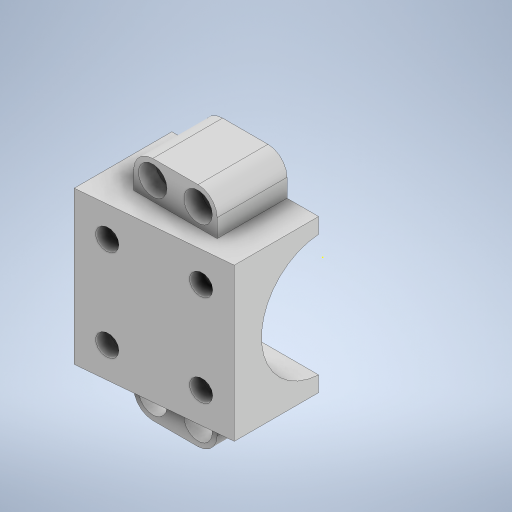
# Autodesk Inventor part: uchwyt
Saved by Autodesk Inventor 2023 (Build 270158000, 158)
## iProperties
Created: 2023-05-30
Part Number: uchwyt
Material: Ogólny
Document SubType Name: Modeling
Designer: Kamil
Density: 1 g/cm^3
Appearance: Domyślna
Author: Kamil
Autodesk Inventor part; units mm, degrees
ref_plane "YZ Plane" through (0, 0, 0) normal (1, 0, 0) x (0, 1, 0)
ref_plane "XZ Plane" through (0, 0, 0) normal (0, 1, 0) x (-1, 0, 0)
ref_plane "XY Plane" through (0, 0, 0) normal (0, 0, 1) x (1, 0, 0)
sketch "Szkic1" plane through (0, 0, 0) normal (0, 1, 0) x (-1, 0, 0)
  line L0 (-115.2766, 10.5) -> (-153.7841, 10.5)
  line L1 (-153.7841, 10.5) -> (-153.7841, 49.5698)
  line L2 (-153.7841, 49.5698) -> (-120, 49.5698)
  line L3 (-113.7841, 10.5) -> (-113.7841, 10.5489)
  line L4 (-19.8138, 58.6953) -> (-19.8138, 1.8047)
  line L5 (-19.8138, 58.6953) -> (-120, 49.5698)
  line L6 (-19.8138, 1.8047) -> (-115.2766, 10.5)
  point P0 (0, 0)
  constraints: 14 end point, 1 horizontal, 1 parallel, 1 perpendicular, 1 point on line, 1 vertical
extrude "Wyciągnięcie proste1" add sketch "Szkic1" along normal blind 40
sketch "Szkic2" plane through (0, 40, 0) normal (0, 1, 0) x (1, 0, 0)
  line L0 (120, -49.5698) -> (153.7841, -49.5698) projected
  line L1 (153.7841, -49.5698) -> (153.7841, -10.5) projected
  line L2 (153.7841, -10.5) -> (115.2766, -10.5) projected
  line L3 (115.2766, -10.5) -> (19.8138, -1.8047) projected
  line L4 (19.8138, -1.8047) -> (19.8138, -58.6953) projected
  line L5 (19.8138, -58.6953) -> (120, -49.5698) projected
  line L6 (19.8138, -30.25) -> (183, -30.25)
  point P0 (0, 0)
  point P1 (153.7841, -30.25)
  constraints: 2 end point, 1 horizontal, 1 midpoint
extrude "Wyciągnięcie proste2" cut sketch "Szkic2" against normal blind 40 contours L6 L4 L3 L2 L1
sketch "Szkic3" plane through (153.7841, 0, 49.5698) normal (1, 0, 0) x (0, 0, -1)
  line L0 (19.3198, 0) -> (19.3198, 40) projected
  line L1 (19.3198, 40) -> (19.3198, 0) projected
  circle A0 centre (19.3198, 20) radius 16
  point P0 (49.5698, 0)
  dimension "d4" = 32
  constraints: 1 centre point, 1 midpoint
  measures "d4" diameter of A0
extrude "Wyciągnięcie proste3" cut sketch "Szkic3" against normal through all
sketch "Szkic4" plane through (0, 40, 0) normal (0, 1, 0) x (1, 0, 0)
  line L0 (19.8138, -30.25) -> (19.8138, -58.6953) projected
  line L1 (19.8138, -30.25) -> (39.8138, -30.25)
  line L2 (39.8138, -30.25) -> (39.8138, -60.25)
  line L3 (39.8138, -60.25) -> (19.8138, -60.25)
  line L4 (19.8138, -60.25) -> (19.8138, -30.25)
  point P0 (0, 0)
  dimension "d7" = 20
  dimension "d8" = 30
  constraints: 8 end point, 2 parallel, 1 horizontal, 1 perpendicular
  measures "d7" distance of L2.end L3.end
  measures "d8" distance of L1.end L2.end
extrude "Wyciągnięcie proste4" cut sketch "Szkic4" against normal through all
sketch "Szkic5" plane through (120, 0, 49.5698) normal (0, 0, 1) x (1, 0, 0)
  line L0 (0, 40) -> (33.7841, 40) projected
  line L1 (0, 0) -> (0, 40) projected
  line L2 (33.7841, 40) -> (-80.1862, 40) projected
  line L3 (33.7841, 40) -> (0, 40)
  line L4 (33.7841, 36) -> (33.7841, 40) projected
  line L5 (33.7841, 40) -> (0, 40)
  line L6 (0, 40) -> (0, 52)
  line L7 (0, 52) -> (33.7841, 52)
  line L8 (33.7841, 52) -> (33.7841, 40)
  line L9 (0, 52) -> (5, 52)
  line L10 (5, 40) -> (0, 40)
  line L11 (0, 40) -> (0, 52)
  line L12 (33.7841, 52) -> (28.7841, 52)
  line L13 (28.7841, 40) -> (33.7841, 40)
  line L14 (33.7841, 40) -> (33.7841, 52)
  circle A0 centre (5, 44.75) radius 2.25
  circle A1 centre (28.7841, 44.75) radius 2.25
  circle A2 centre (16.8921, 44.75) radius 2.25
  circle A3 centre (5, 44.75) radius 5
  circle A4 centre (28.7841, 44.75) radius 5
  line L15 (5, 49.75) -> (28.7841, 49.75)
  point P0 (-120, 0)
  point P1 (0, 44.75)
  point P2 (33.7841, 44.75)
  dimension "d12" = 12
  dimension "d13" = 5
  dimension "d14" = 5
  constraints: 24 end point, 4 horizontal, 4 parallel, 3 centre point, 2 coincident, 2 point on line, 2 vertical, 1 collinear, 1 perpendicular, 6 other
  measures "d12" distance of L5.end L6.end
  measures "d13" distance of L10.start L10.end
  measures "d14" distance of L13.end L13.start
extrude "Wyciągnięcie proste5" add sketch "Szkic5" against normal up to surface (19.3198 mm away) contours L6 A3 L0 | A3 L0 | A3 L15 A4 L0 | A4 L0 | A4 L8 L0 picked at (4.3892, 40.8388) picked at (28.1733, 40.8388)
sketch "Szkic6" plane through (120, 0, 49.5698) normal (0, 0, 1) x (1, 0, 0)
  circle A0 centre (28.7841, 44.75) radius 2.25 projected
  circle A1 centre (16.8921, 44.75) radius 2.25 projected
  circle A2 centre (5, 44.75) radius 2.25 projected
  line L0 (0, 0) -> (33.7841, 0) projected
  line L1 (33.7841, 0) -> (33.7841, 44.75) projected
  arc A3 (33.7841, 44.75) -> (28.7841, 49.75) centre (28.7841, 44.75) ccw projected
  line L2 (28.7841, 49.75) -> (5, 49.75) projected
  arc A4 (5, 49.75) -> (0, 44.75) centre (5, 44.75) ccw projected
  line L3 (0, 44.75) -> (0, 40) projected
  line L4 (0, 0) -> (0, 40) projected
  line L5 (0, 40) -> (-80.1862, 40) projected
  line L6 (0, 40) -> (0, 0)
  line L7 (-80.1862, 0) -> (33.7841, 0) projected
  line L8 (0, 20) -> (40, 20)
  circle A5 centre (28.7841, -4.75) radius 2.25
  circle A6 centre (16.8921, -4.75) radius 2.25
  circle A7 centre (5, -4.75) radius 2.25
  line L9 (33.7841, 40) -> (33.7841, -4.75)
  arc A8 (28.7841, -9.75) -> (33.7841, -4.75) centre (28.7841, -4.75) ccw
  line L10 (28.7841, -9.75) -> (5, -9.75)
  arc A9 (0, -4.75) -> (5, -9.75) centre (5, -4.75) ccw
  line L11 (0, -4.75) -> (0, 0)
  point P0 (-120, 0)
  constraints: 10 end point, 10 symmetric about line, 5 centre point, 4 point on circle, 1 horizontal, 1 midpoint, 1 perpendicular, 5 other
extrude "Wyciągnięcie proste6" add sketch "Szkic6" against normal up to surface (19.3198 mm away) contours L0 L9 A8 L10 A9 L11
sketch "Szkic7" plane through (125, 49.75, 49.5698) normal (0, 0, 1) x (1, 0, 0)
  circle A0 centre (0, -54.5) radius 2.25 projected
  circle A1 centre (23.7841, -54.5) radius 2.25 projected
  circle A2 centre (11.8921, -54.5) radius 2.25 projected
  circle A3 centre (23.7841, -5) radius 2.25 projected
  circle A4 centre (11.8921, -5) radius 2.25 projected
  circle A5 centre (0, -5) radius 2.25 projected
  line L0 (28.7841, -54.5) -> (28.7841, -5) projected
  arc A6 (28.7841, -5) -> (23.7841, 0) centre (23.7841, -5) ccw projected
  line L1 (23.7841, 0) -> (0, 0) projected
  arc A7 (0, 0) -> (-5, -5) centre (0, -5) ccw projected
  line L2 (-5, -5) -> (-5, -9.75) projected
  line L3 (-5, -49.75) -> (-5, -9.75) projected
  line L4 (-5, -49.75) -> (-5, -54.5) projected
  arc A8 (-5, -54.5) -> (0, -59.5) centre (0, -54.5) ccw projected
  line L5 (0, -59.5) -> (23.7841, -59.5) projected
  arc A9 (23.7841, -59.5) -> (28.7841, -54.5) centre (23.7841, -54.5) ccw projected
  point P0 (-125, -49.75)
hole "Otwór1" at (125, 44.75, 49.5698) at (136.8921, 44.75, 49.5698) at (148.7841, 44.75, 49.5698) at (148.7841, -4.75, 49.5698) at (136.8921, -4.75, 49.5698) at (125, -4.75, 49.5698) direction (0, 0, -1) diameter 4.5 depth 40 tip angle 118 counterbore diameter 7.5 counterbore depth 4.5
sketch "Szkic8" plane through (125, 49.75, 49.5698) normal (0, 0, 1) x (1, 0, 0)
  circle A0 centre (11.8921, -54.5) radius 3.75 projected
  circle A1 centre (23.7841, -5) radius 3.75 projected
  circle A2 centre (0, -5) radius 3.75 projected
  circle A3 centre (11.8921, -5) radius 3.75 projected
  circle A4 centre (23.7841, -54.5) radius 3.75 projected
  circle A5 centre (0, -54.5) radius 3.75 projected
  line L0 (28.7841, -54.5) -> (28.7841, -5) projected
  arc A6 (28.7841, -5) -> (23.7841, 0) centre (23.7841, -5) ccw projected
  line L1 (23.7841, 0) -> (0, 0) projected
  arc A7 (0, 0) -> (-5, -5) centre (0, -5) ccw projected
  line L2 (-5, -5) -> (-5, -9.75) projected
  line L3 (-5, -49.75) -> (-5, -9.75) projected
  line L4 (-5, -49.75) -> (-5, -54.5) projected
  arc A8 (-5, -54.5) -> (0, -59.5) centre (0, -54.5) ccw projected
  line L5 (0, -59.5) -> (23.7841, -59.5) projected
  arc A9 (23.7841, -59.5) -> (28.7841, -54.5) centre (23.7841, -54.5) ccw projected
  line L6 (-85.1862, -9.75) -> (-85.1862, -49.75) projected
  circle A10 centre (0, -5) radius 2.25 projected
  line L7 (0, -5) -> (-30, -5)
  line L8 (-30, -5) -> (-30, -64)
  circle A11 centre (0, -54.5) radius 2.25 projected
  circle A12 centre (11.8921, -5) radius 2.25 projected
  circle A13 centre (11.8921, -54.5) radius 2.25 projected
  arc A14 (-55, -5) -> (-60, 0) centre (-60, -5) ccw
  line L9 (-55, -5) -> (-55, -9.75)
  line L10 (-55, -49.75) -> (-55, -9.75)
  line L11 (-55, -49.75) -> (-55, -54.5)
  arc A15 (-60, -59.5) -> (-55, -54.5) centre (-60, -54.5) ccw
  line L12 (-60, -59.5) -> (-71.8921, -59.5)
  arc A16 (-71.8921, 0) -> (-76.8921, -5) centre (-71.8921, -5) ccw
  arc A17 (-76.8921, -54.5) -> (-71.8921, -59.5) centre (-71.8921, -54.5) ccw
  line L13 (-76.8921, -5) -> (-76.8921, -54.5)
  line L14 (-71.8921, 0) -> (-60, 0)
  point P0 (-125, -49.75)
  point P1 (-83.7841, -59.5)
  dimension "d28" = 30
  constraints: 16 end point, 9 symmetric about line, 8 point on circle, 4 centre point, 3 tangent, 2 horizontal, 1 perpendicular, 2 other
  measures "d28" distance of L7.start L7.end
extrude "Wyciągnięcie proste7" add sketch "Szkic8" against normal up to surface (19.3198 mm away) contours L9 L10 L11 A15 L12 A17 L13 A16 L14 A14
sketch "Szkic9" plane through (125, 49.75, 49.5698) normal (0, 0, 1) x (1, 0, 0)
  line L0 (-55, -9.75) -> (-76.8921, -9.75) projected
  line L1 (-55, -9.75) -> (-55, -5) projected
  arc A0 (-55, -5) -> (-60, 0) centre (-60, -5) ccw projected
  line L2 (-60, 0) -> (-71.8921, 0) projected
  arc A1 (-71.8921, 0) -> (-76.8921, -5) centre (-71.8921, -5) ccw projected
  line L3 (-76.8921, -5) -> (-76.8921, -9.75) projected
  line L4 (-76.8921, -49.75) -> (-55, -49.75) projected
  line L5 (-76.8921, -49.75) -> (-76.8921, -54.5) projected
  arc A2 (-76.8921, -54.5) -> (-71.8921, -59.5) centre (-71.8921, -54.5) ccw projected
  line L6 (-71.8921, -59.5) -> (-60, -59.5) projected
  arc A3 (-60, -59.5) -> (-55, -54.5) centre (-60, -54.5) ccw projected
  line L7 (-55, -54.5) -> (-55, -49.75) projected
  point P0 (-125, -49.75)
hole "Otwór2" at (53.1079, 44.75, 49.5698) at (65, 44.75, 49.5698) at (53.1079, -4.75, 49.5698) at (65, -4.75, 49.5698) direction (0, 0, -1) diameter 4.5 depth 40 tip angle 118 counterbore diameter 7.5 counterbore depth 4.5
sketch "Szkic10" plane through (48.1079, 20, 30.25) normal (-1, 0, 0) x (0, 0, 1)
  point P0 (-30.25, -20)
sketch "Szkic11" plane through (48.1079, 20, 30.25) normal (-1, 0, 0) x (0, 0, 1)
  arc A0 (0, -16) -> (0, 16) centre (0, 0) ccw projected
  line L0 (0, -16) -> (0, 16) projected
  point P0 (-30.25, -20)
extrude "Wyciągnięcie proste8" cut sketch "Szkic11" against normal through all
sketch "Szkic12" plane through (153.7841, 36, 30.25) normal (0, 0, -1) x (-1, 0, 0)
  circle A0 centre (100.6762, 8.75) radius 2.25 projected
  circle A1 centre (88.7841, 8.75) radius 2.25 projected
  line L0 (0, 0) -> (113.9703, 0) projected
  line L1 (113.9703, 0) -> (113.9703, 4) projected
  line L2 (105.6762, 4) -> (113.9703, 4) projected
  line L3 (105.6762, 4) -> (105.6762, 8.75) projected
  arc A2 (105.6762, 8.75) -> (100.6762, 13.75) centre (100.6762, 8.75) ccw projected
  line L4 (100.6762, 13.75) -> (88.7841, 13.75) projected
  arc A3 (88.7841, 13.75) -> (83.7841, 8.75) centre (88.7841, 8.75) ccw projected
  line L5 (83.7841, 8.75) -> (83.7841, 4) projected
  line L6 (33.7841, 4) -> (83.7841, 4) projected
  line L7 (33.7841, 4) -> (33.7841, 8.75) projected
  arc A4 (33.7841, 8.75) -> (28.7841, 13.75) centre (28.7841, 8.75) ccw projected
  line L8 (28.7841, 13.75) -> (5, 13.75) projected
  arc A5 (5, 13.75) -> (0, 8.75) centre (5, 8.75) ccw projected
  line L9 (0, 0) -> (0, 8.75) projected
  circle A6 centre (28.7841, 8.75) radius 2.25 projected
  circle A7 centre (16.8921, 8.75) radius 2.25 projected
  circle A8 centre (5, 8.75) radius 2.25 projected
  line L10 (88.7841, 13.75) -> (100.6762, 13.75) projected
  line L11 (94.7302, 13.75) -> (94.7302, -45.75)
  line L12 (100.6762, -45.75) -> (88.7841, -45.75) projected
  line L13 (83.7841, 4) -> (75.49, 4)
  line L14 (75.49, 4) -> (75.49, -45.75)
  line L15 (83.7841, -36) -> (33.7841, -36) projected
  arc A9 (83.7841, -40.75) -> (88.7841, -45.75) centre (88.7841, -40.75) ccw projected
  line L16 (83.7841, -36) -> (83.7841, -40.75) projected
  line L17 (33.7841, -40.75) -> (33.7841, -36) projected
  line L18 (33.7841, 4) -> (33.7841, -36)
  point P0 (153.7841, -36)
  point P1 (75.49, -36)
  point P2 (75.49, 4)
  constraints: 8 end point, 2 midpoint, 1 symmetric about line, 1 vertical
extrude "Wyciągnięcie proste9" cut sketch "Szkic12" against normal through all contours L18 L6 L14 L0 | L0 L14 L15 L18
sketch "Szkic13" plane through (39.8138, 0, 56.8735) normal (0.0907098, 0, 0.9958774) x (0.9958774, 0, -0.0907098)
  line L0 (38.6396, 0) -> (38.6396, 40) projected
  line L1 (0, 40) -> (38.6396, 40) projected
  line L2 (0, 40) -> (0, 0) projected
  line L3 (0, 0) -> (38.6396, 0) projected
  line L4 (0, 40) -> (8, 40)
  line L5 (8, 40) -> (8, 32)
  line L6 (8, 32) -> (0, 32)
  line L7 (0, 32) -> (0, 40)
  line L8 (38.6396, 40) -> (30.6396, 40)
  line L9 (30.6396, 40) -> (30.6396, 32)
  line L10 (30.6396, 32) -> (38.6396, 32)
  line L11 (38.6396, 32) -> (38.6396, 40)
  line L12 (38.6396, 0) -> (30.6396, 0)
  line L13 (30.6396, 0) -> (30.6396, 8)
  line L14 (30.6396, 8) -> (38.6396, 8)
  line L15 (38.6396, 8) -> (38.6396, 0)
  line L16 (0, 0) -> (8, 0)
  line L17 (8, 0) -> (8, 8)
  line L18 (8, 8) -> (0, 8)
  line L19 (0, 8) -> (0, 0)
  point P0 (-34.4907, 0)
  dimension "d42" = 8
  dimension "d43" = 8
  dimension "d44" = 8
  dimension "d45" = 8
  dimension "d46" = 8
  dimension "d47" = 8
  dimension "d48" = 8
  dimension "d49" = 8
  constraints: 32 end point, 8 parallel, 5 coincident, 4 horizontal, 4 perpendicular
  measures "d42" distance of L5.end L6.end
  measures "d43" distance of L4.end L5.end
  measures "d44" distance of L10.end L9.end
  measures "d45" distance of L9.end L8.end
  measures "d46" distance of L13.end L14.end
  measures "d47" distance of L12.end L13.end
  measures "d48" distance of L18.end L17.end
  measures "d49" distance of L17.end L16.end
hole "Otwór3" at (47.7808, 32, 56.1479) at (70.3271, 32, 54.0942) at (47.7808, 8, 56.1479) at (70.3271, 8, 54.0942) direction (-0.0907098, 0, -0.9958774) diameter 4.5 end through all counterbore diameter 5.6 counterbore depth 4
sketch "Szkic14" plane through (125, 49.75, 49.5698) normal (0, 0, 1) x (1, 0, 0)
  line L0 (-85.1862, -9.75) -> (-46.7059, -9.75) projected
  line L1 (-85.1862, -49.75) -> (-46.7059, -49.75) projected
  circle A0 centre (11.8921, -54.5) radius 3.75 projected
  circle A1 centre (23.7841, -5) radius 3.75 projected
  circle A2 centre (0, -5) radius 3.75 projected
  circle A3 centre (11.8921, -5) radius 3.75 projected
  circle A4 centre (23.7841, -54.5) radius 3.75 projected
  circle A5 centre (0, -54.5) radius 3.75 projected
  line L2 (28.7841, -54.5) -> (28.7841, -5) projected
  arc A6 (28.7841, -5) -> (23.7841, 0) centre (23.7841, -5) ccw projected
  line L3 (23.7841, 0) -> (0, 0) projected
  arc A7 (0, 0) -> (-5, -5) centre (0, -5) ccw projected
  line L4 (-5, -5) -> (-5, -54.5) projected
  arc A8 (-5, -54.5) -> (0, -59.5) centre (0, -54.5) ccw projected
  line L5 (0, -59.5) -> (23.7841, -59.5) projected
  arc A9 (23.7841, -59.5) -> (28.7841, -54.5) centre (23.7841, -54.5) ccw projected
  line L6 (-5, -9.75) -> (28.7841, -9.75)
  line L7 (28.7841, -9.75) -> (28.7841, -49.75)
  line L8 (28.7841, -49.75) -> (-5, -49.75)
  line L9 (-5, -49.75) -> (-5, -9.75)
  line L10 (-5, -9.75) -> (3, -9.75)
  line L11 (3, -9.75) -> (3, -17.75)
  line L12 (3, -17.75) -> (-5, -17.75)
  line L13 (-5, -17.75) -> (-5, -9.75)
  line L14 (28.7841, -9.75) -> (13.7841, -9.75)
  line L15 (13.7841, -9.75) -> (13.7841, -17.75)
  line L16 (13.7841, -17.75) -> (28.7841, -17.75)
  line L17 (28.7841, -17.75) -> (28.7841, -9.75)
  line L18 (-5, -49.75) -> (3, -49.75)
  line L19 (3, -49.75) -> (3, -41.75)
  line L20 (3, -41.75) -> (-5, -41.75)
  line L21 (-5, -41.75) -> (-5, -49.75)
  line L22 (28.7841, -49.75) -> (13.7841, -49.75)
  line L23 (13.7841, -49.75) -> (13.7841, -41.75)
  line L24 (13.7841, -41.75) -> (28.7841, -41.75)
  line L25 (28.7841, -41.75) -> (28.7841, -49.75)
  point P0 (-125, -49.75)
  dimension "d57" = 8
  dimension "d58" = 8
  dimension "d59" = 15
  dimension "d60" = 8
  dimension "d61" = 8
  constraints: 40 end point, 10 parallel, 5 horizontal, 5 perpendicular, 5 point on line, 4 coincident
  measures "d57" distance of L11.end L12.end
  measures "d58" distance of L10.end L11.end
  measures "d59" distance of L16.end L15.end
  measures "d60" distance of L15.end L14.end
  measures "d61" distance of L19.end L18.end
hole "Otwór4" at (128, 32, 49.5698) at (138.7841, 32, 49.5698) at (138.7841, 8, 49.5698) at (128, 8, 49.5698) direction (0, 0, -1) diameter 4.5 end through all counterbore diameter 5.6 counterbore depth 4
sketch "Szkic15" plane through (153.7841, 36, 30.25) normal (0, 0, -1) x (-1, 0, 0)
  line L0 (33.7841, 0) -> (33.7841, 8.75) projected
  arc A0 (33.7841, 8.75) -> (28.7841, 13.75) centre (28.7841, 8.75) ccw projected
  line L1 (28.7841, 13.75) -> (5, 13.75) projected
  arc A1 (5, 13.75) -> (0, 8.75) centre (5, 8.75) ccw projected
  line L2 (0, 0) -> (0, 8.75) projected
  line L3 (0, 0) -> (33.7841, 0) projected
  circle A2 centre (28.7841, 8.75) radius 2.25 projected
  circle A3 centre (16.8921, 8.75) radius 2.25 projected
  circle A4 centre (5, 8.75) radius 2.25 projected
  line L4 (33.7841, -40.75) -> (33.7841, -32) projected
  line L5 (33.7841, -32) -> (0, -32) projected
  line L6 (0, -32) -> (0, -40.75) projected
  arc A5 (0, -40.75) -> (5, -45.75) centre (5, -40.75) ccw projected
  line L7 (5, -45.75) -> (28.7841, -45.75) projected
  arc A6 (28.7841, -45.75) -> (33.7841, -40.75) centre (28.7841, -40.75) ccw projected
  circle A7 centre (28.7841, -40.75) radius 2.25 projected
  circle A8 centre (5, -40.75) radius 2.25 projected
  circle A9 centre (16.8921, -40.75) radius 2.25 projected
  line L8 (75.49, 4) -> (75.49, 0) projected
  line L9 (75.49, 0) -> (113.9703, 0) projected
  line L10 (113.9703, 0) -> (113.9703, 4) projected
  line L11 (105.6762, 4) -> (113.9703, 4) projected
  line L12 (105.6762, 4) -> (105.6762, 8.75) projected
  arc A10 (105.6762, 8.75) -> (100.6762, 13.75) centre (100.6762, 8.75) ccw projected
  line L13 (100.6762, 13.75) -> (88.7841, 13.75) projected
  arc A11 (88.7841, 13.75) -> (83.7841, 8.75) centre (88.7841, 8.75) ccw projected
  line L14 (83.7841, 8.75) -> (83.7841, 4) projected
  line L15 (75.49, 4) -> (83.7841, 4) projected
  circle A12 centre (88.7841, 8.75) radius 2.25 projected
  circle A13 centre (100.6762, 8.75) radius 2.25 projected
  circle A14 centre (88.7841, -40.75) radius 2.25 projected
  circle A15 centre (100.6762, -40.75) radius 2.25 projected
  line L16 (75.49, -32) -> (75.49, -36) projected
  line L17 (83.7841, -36) -> (75.49, -36) projected
  line L18 (83.7841, -36) -> (83.7841, -40.75) projected
  arc A16 (83.7841, -40.75) -> (88.7841, -45.75) centre (88.7841, -40.75) ccw projected
  line L19 (88.7841, -45.75) -> (100.6762, -45.75) projected
  arc A17 (100.6762, -45.75) -> (105.6762, -40.75) centre (100.6762, -40.75) ccw projected
  line L20 (105.6762, -40.75) -> (105.6762, -36) projected
  line L21 (113.9703, -36) -> (105.6762, -36) projected
  line L22 (113.9703, -36) -> (113.9703, -32) projected
  line L23 (113.9703, -32) -> (75.49, -32) projected
  line L24 (0, 0) -> (33.7841, 0)
  line L25 (33.7841, 0) -> (33.7841, -32)
  line L26 (33.7841, -32) -> (0, -32)
  line L27 (0, -32) -> (0, 0)
  line L28 (75.49, 0) -> (113.9703, 0)
  line L29 (113.9703, 0) -> (113.9703, -32)
  line L30 (113.9703, -32) -> (75.49, -32)
  line L31 (75.49, -32) -> (75.49, 0)
  point P0 (153.7841, -36)
  constraints: 16 end point, 4 parallel, 2 horizontal, 2 perpendicular
extrude "Wyciągnięcie proste10" cut sketch "Szkic15" against normal blind 1 contours L3 L2 A1 L1 A0 L0 | L25 L5 L27 L3 | L4 A6 L7 A5 L6 L5 | A2 | A3 | A4 | A7 | A8 | A9 | L15 L14 A11 L13 A10 L12 L11 L10 L9 L8 | L9 L29 L23 L31 | L23 L22 L21 L20 A17 L19 A16 L18 L17 L16
sketch "Szkic16" plane through (125, 49.75, 49.5698) normal (0, 0, 1) x (1, 0, 0)
  line L0 (-15, 12) -> (49, 12)
  line L1 (49, 12) -> (49, -79)
  line L2 (49, -79) -> (-15, -79)
  line L3 (-15, -79) -> (-15, 12)
  point P0 (-125, -49.75)
  constraints: 8 end point, 2 parallel, 1 horizontal, 1 perpendicular
extrude "Wyciągnięcie proste11" cut sketch "Szkic16" against normal through all
